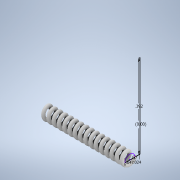
# Autodesk Inventor part: Part1
Saved by Autodesk Inventor 2020 (Build 240168000, 168)
## iProperties
Created: 2019-07-08
Part Number: Part1
Material: Generic
Document SubType Name: Modeling
Designer: ColinP
Density: 1 g/cm^3
Appearance: Default
Author: ColinP
Autodesk Inventor part; units mm, degrees
ref_plane "YZ Plane" through (0, 0, 0) normal (1, 0, 0) x (0, 1, 0)
ref_plane "XZ Plane" through (0, 0, 0) normal (0, 1, 0) x (-1, 0, 0)
ref_plane "XY Plane" through (0, 0, 0) normal (0, 0, 1) x (1, 0, 0)
sketch "Sketch1" plane through (0, 0, 0) normal (0, 1, 0) x (-1, 0, 0)
  circle A0 centre (0, 0) radius 0.1905
  dimension "d0" = 0.381
  constraints: 1 centre point, 1 coincident
  measures "d0" diameter of A0
sketch "Sketch2" plane through (0, 0, 0) normal (0, 0, 1) x (1, 0, 0)
  point P0 (0, 0)
sketch "Sketch3" plane through (0, 0, 0) normal (1, 0, 0) x (0, 1, 0)
  line L0 (0, 0) -> (0, -0.5969)
  line L1 (0, -0.5969) -> (9.9568, -0.5969)
  line L2 (0, -0.5969) -> (9.9568, -0.5969) construction
  dimension "d1" = 0.5969
  dimension "d2" = 9.9568
  dimension "d3" = 0
  constraints: 6 end point, 2 horizontal, 1 collinear, 1 vertical
  measures "d1" distance of L0.start L0.end
  measures "d2" distance of L0.end L1.end
  measures "d3" distance between parallel lines of L1 L2
sketch "Sketch4" plane through (0, 0, 0) normal (0, 1, 0) x (-1, 0, 0)
  line L0 (0, 0) -> (0, 0.5969)
  line L1 (0, 0.5969) -> (9.9568, 0.5969)
  dimension "d4" = 0.5969
  dimension "d5" = 9.9568
  dimension "d6" = 90
  constraints: 4 end point, 1 perpendicular, 1 vertical
  measures "d4" distance of L0.start L0.end
  measures "d5" distance of L0.end L1.end
  measures "d6" angle of L0 L1
coil "Coil1" sketch "Sketch1" operation add axis through (0, 0, 0.5969) along (-1, 0, 0) pitch 0.6223 turns 16 hand right
sketch "Sketch5" plane through (0, 0, 0) normal (1, 0, 0) x (0, 1, 0)
  line L0 (0, 0) -> (0, 1.1938)
  arc A0 (0, 0) -> (0, 1.1938) centre (0.0053, 0.5969) ccw
  dimension "d15" = 1.1938
  constraints: 2 end point, 2 point on circle, 1 centre point, 1 vertical
  measures "d15" distance of L0.start L0.end
body "Solid1"
